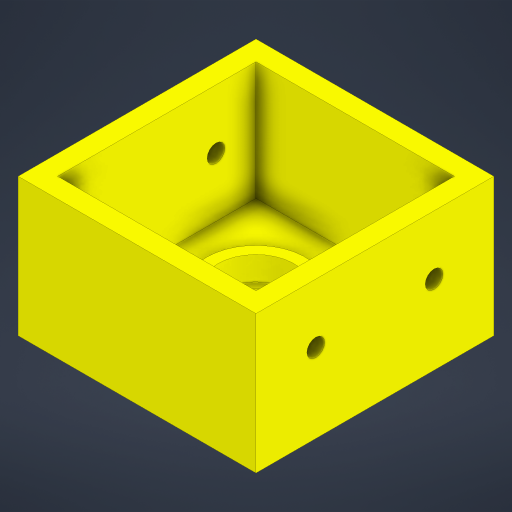
# Autodesk Inventor part: Part18
Saved by Autodesk Inventor 2023 (Build 270158000, 158)
## iProperties
Created: 2023-08-13
Part Number: Part18
Material: PBT Plastic
Document SubType Name: Modeling
Designer: Abhinav
Density: 1.31 g/cm^3
Appearance: Default(1)
Mass: 67.9789 g
Surface Area: 240.762 cm^2
Volume: 51.8923 cm^3
Author: Abhinav
Autodesk Inventor part; units mm, degrees
ref_plane "YZ Plane" through (0, 0, 0) normal (1, 0, 0) x (0, 1, 0)
ref_plane "XZ Plane" through (0, 0, 0) normal (0, 1, 0) x (-1, 0, 0)
ref_plane "XY Plane" through (0, 0, 0) normal (0, 0, 1) x (1, 0, 0)
sketch "Sketch1" plane through (0, 0, 0) normal (0, 1, 0) x (-1, 0, 0)
  line L0 (25.15, 25.15) -> (-25.15, 25.15)
  line L1 (-25.15, 25.15) -> (-25.15, -25.15)
  line L2 (-25.15, -25.15) -> (25.15, -25.15)
  line L3 (25.15, -25.15) -> (25.15, 25.15)
  line L4 (25.15, 25.15) -> (-25.15, -25.15) construction
  line L5 (-25.15, 25.15) -> (25.15, -25.15) construction
  line L6 (30.15, 30.15) -> (-30.15, 30.15)
  line L7 (-30.15, 30.15) -> (-30.15, -30.15)
  line L8 (-30.15, -30.15) -> (30.15, -30.15)
  line L9 (30.15, -30.15) -> (30.15, 30.15)
  line L10 (30.15, 30.15) -> (-30.15, -30.15) construction
  line L11 (-30.15, 30.15) -> (30.15, -30.15) construction
  circle A0 centre (0, 0) radius 7.5
  circle A1 centre (0, 0) radius 9.65
  circle A2 centre (0, 0) radius 12.5
  line L12 (0, 0) -> (25.15, 0) construction
  line L13 (0, 0) -> (0, -25.15) construction
  dimension "d1" = 50.3
  dimension "d3" = 60.3
  dimension "d8" = 15
  dimension "d9" = 19.3
  dimension "d10" = 25
  constraints: 28 end point, 6 midpoint, 4 parallel, 4 perpendicular, 3 centre point, 3 coincident, 2 horizontal
  measures "d1" distance of L1.end L0.end
  measures "d3" distance of L7.end L6.end
  measures "d8" diameter of A0
  measures "d9" diameter of A1
  measures "d10" diameter of A2
extrude "Extrusion1" add sketch "Sketch1" along normal blind 30 contours L9 L8 L7 L6
extrude "Extrusion2" add sketch "Sketch1" against normal blind 5 contours L3 L2 L1 L0 | L9 L8 L7 L6 | A1 | A2
extrude "Extrusion3" add sketch "Sketch1" along normal blind 6 contours A2
sketch "Sketch2" plane through (-30.15, 30, -30.15) normal (-1, 0, 0) x (0, 0, 1)
  line L0 (60.3, 0) -> (60.3, -35) construction
  line L1 (0, -35) -> (0, 0) construction
  circle A0 centre (45.15, -15) radius 2.25
  line L2 (30.15, -15) -> (45.15, -15) construction
  line L3 (30.15, -15) -> (15.15, -15) construction
  circle A1 centre (15.15, -15) radius 2.25
  line L4 (60.3, 0) -> (0, 0)
  line L5 (0, 0) -> (0, -30)
  line L6 (0, -30) -> (60.3, -30)
  line L7 (60.3, -30) -> (60.3, 0)
  line L8 (60.3, 0) -> (0, -30) construction
  line L9 (30.15, -15) -> (25.1861, -9.3551) construction
  point P0 (30.15, -30)
  dimension "d13" = 4.5
  dimension "d16" = 15
  dimension "d17" = 15
  dimension "d18" = 4.5
  dimension "d19" = 30
  constraints: 16 end point, 2 centre point, 2 horizontal, 2 parallel, 2 point on line, 1 coincident, 1 midpoint, 1 perpendicular
  measures "d13" diameter of A0
  measures "d16" distance of L2.start L2.end
  measures "d17" distance of L3.start L3.end
  measures "d18" diameter of A1
  measures "d19" distance of L5.end L4.end
extrude "Extrusion4" cut sketch "Sketch2" against normal blind 65 contours A0 | A1
body "Solid1"
